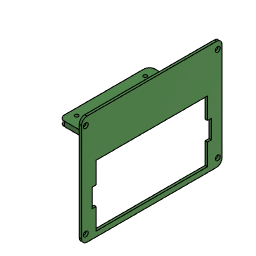
laser_module_power_control_mount v2 (Autodesk Fusion 360 design; units mm, degrees)
Autodesk Fusion 360 part; units mm, degrees
sketch "Sketch1" plane through (0, 0, 0) normal (1, 0, 0) x (0, 1, 0)
  line L0 (45, 35) -> (-45, 35)
  line L1 (-45, 35) -> (-45, -35)
  line L2 (-45, -35) -> (45, -35)
  line L3 (45, -35) -> (45, 35)
  line L4 (45, 35) -> (-45, -35) construction
  line L5 (-45, 35) -> (45, -35) construction
  line L6 (0, 0) -> (0, -35) construction
  line L7 (39.5, 9.4262) -> (-39.5, 9.4262) construction
  line L8 (-39.5, 9.4262) -> (-39.5, -33.5738) construction
  line L9 (-39.5, -33.5738) -> (39.5, -33.5738) construction
  line L10 (39.5, -33.5738) -> (39.5, 9.4262) construction
  line L11 (39.5, 9.4262) -> (-39.5, -33.5738) construction
  line L12 (-39.5, 9.4262) -> (39.5, -33.5738) construction
  line L13 (35.7, 7.5762) -> (-35.7, 7.5762)
  line L14 (-35.7, 7.5762) -> (-35.7, -31.7238)
  line L15 (-35.7, -31.7238) -> (35.7, -31.7238)
  line L16 (35.7, -31.7238) -> (35.7, 7.5762)
  line L17 (35.7, 7.5762) -> (-35.7, -31.7238) construction
  line L18 (-35.7, 7.5762) -> (35.7, -31.7238) construction
  circle A0 centre (42.2913, -30.0813) radius 1.575
  line L19 (0, 0) -> (10.5805, 0) construction
  circle A1 centre (-42.2913, -30.0813) radius 1.575
  circle A2 centre (42.2913, 30.0813) radius 1.575
  circle A3 centre (-42.2913, 30.0813) radius 1.575
  line L20 (0, 0) -> (0, 0.8708) construction
  line L21 (0, 0.8708) -> (0, 35) construction
  line L22 (25, 32.3854) -> (-25, 32.3854) construction
  line L23 (-25, 32.3854) -> (-25, 12.3854) construction
  line L24 (-25, 12.3854) -> (25, 12.3854) construction
  line L25 (25, 12.3854) -> (25, 32.3854) construction
  line L26 (25, 32.3854) -> (-25, 12.3854) construction
  line L27 (-25, 32.3854) -> (25, 12.3854) construction
  line L28 (29, 12.3854) -> (-29, 12.3854)
  line L29 (-29, 12.3854) -> (-29, 9.3854)
  line L30 (-29, 9.3854) -> (29, 9.3854)
  line L31 (29, 9.3854) -> (29, 12.3854)
  line L32 (29, 12.3854) -> (-29, 9.3854) construction
  line L33 (-29, 12.3854) -> (29, 9.3854) construction
  line L34 (0, -12.0738) -> (39.5, -12.0738) construction
  line L35 (35.7, -6.0738) -> (38.2, -6.0738)
  line L36 (38.2, -6.0738) -> (38.2, -18.0738)
  line L37 (38.2, -18.0738) -> (35.7, -18.0738)
  line L38 (35.7, -18.0738) -> (35.7, -6.0738)
  line L39 (-38.2, -18.0738) -> (-35.7, -18.0738)
  line L40 (-38.2, -6.0738) -> (-38.2, -18.0738)
  line L41 (-35.7, -6.0738) -> (-38.2, -6.0738)
  point P0 (0, -12.0738)
  point P1 (0, -12.0738)
  point P2 (0, 22.3854)
  point P3 (0, 10.8854)
  point P4 (38.2, -12.0738)
  dimension "d8" = 90
  dimension "d9" = 70
  dimension "d12" = 79
  dimension "d13" = 43
  dimension "d14" = 71.4
  dimension "d15" = 39.3
  dimension "d17" = 3.15
  dimension "d21" = 50
  dimension "d22" = 20
  dimension "d25" = 58
  dimension "d26" = 3
  dimension "d58" = 2.5
  dimension "d59" = 12
  constraint horizontal L0
  constraint perpendicular L0 L1
  constraint parallel L0 L2
  constraint parallel L1 L3
  constraint coincident L4 L6.start
  constraint coincident L5 L6.start
  constraint coincident L6.start L19.start
  constraint vertical L6
  constraint midpoint L2 L6.end
  constraint horizontal L7
  constraint perpendicular L7 L8
  constraint parallel L7 L9
  constraint parallel L8 L10
  constraint coincident L11 P1
  constraint coincident L12 P1
  constraint coincident L6 P1
  constraint horizontal L13
  constraint perpendicular L13 L14
  constraint parallel L13 L15
  constraint parallel L14 L16
  constraint coincident L17 P1
  constraint coincident L18 P1
  constraint coincident P1 P0
  constraint perpendicular L6 L19
  constraint symmetric L6 A0 A1
  constraint symmetric A0 L19 A2
  constraint symmetric L19 A1 A3
  constraint perpendicular L19 L20
  constraint midpoint L0 L21.end
  constraint perpendicular L0 L21
  constraint horizontal L22
  constraint perpendicular L22 L23
  constraint parallel L22 L24
  constraint parallel L23 L25
  constraint coincident L26 P2
  constraint coincident L27 P2
  constraint coincident L21 P2
  constraint horizontal L28
  constraint perpendicular L28 L29
  constraint parallel L28 L30
  constraint parallel L29 L31
  constraint coincident L32 P3
  constraint coincident L33 P3
  constraint coincident L21 P3
  constraint coincident L23.end L28
  constraint horizontal L34
  constraint midpoint L10 L34.end
  constraint horizontal L35
  constraint vertical L36
  constraint horizontal L37
  constraint vertical L38
  constraint coincident L16 L35.start
  constraint midpoint L36 P4
  constraint coincident L34 P4
  constraint symmetric L6 L35.start L41.start
  constraint symmetric L6 L35.end L40.start
  constraint symmetric L6 L36.end L39.start
  constraint symmetric L6 L37.end L39.end
  measures "d8" distance of L1.end L2.end
  measures "d9" distance of L0.end L1.end
  measures "d12" distance of L8.end L9.end
  measures "d13" distance of L7.end L8.end
  measures "d14" distance of L14.end L15.end
  measures "d15" distance of L13.end L14.end
  measures "d17" diameter of A0
  measures "d21" distance of L23.end L24.end
  measures "d22" distance of L22.end L23.end
  measures "d25" distance of L29.end L30.end
  measures "d26" distance of L28.end L29.end
  measures "d58" distance of L35.start L35.end
  measures "d59" distance of L35.start L37.end
extrude "Extrude1" add sketch "Sketch1" along normal blind 1.5 contours L0 L1 L2 L3 | L28 L29 L30 L31
extrude "Extrude2" add sketch "Sketch1" against normal blind 29 contours L28 L29 L30 L31
sketch "Sketch2" plane through (0, 0, 12.3854) normal (0, 0, 1) x (-1, 0, 0)
  line L0 (0, 29) -> (0, -29)
  line L1 (0, -29) -> (29, -29)
  line L2 (29, -29) -> (29, 29)
  line L3 (29, 29) -> (0, 29)
  line L4 (0, 29) -> (29, -29) construction
  line L5 (27.5, 25) -> (1.5, 25) construction
  line L6 (1.5, 25) -> (1.5, -25) construction
  line L7 (1.5, -25) -> (27.5, -25) construction
  line L8 (27.5, -25) -> (27.5, 25) construction
  line L9 (27.5, 25) -> (1.5, -25) construction
  line L10 (1.5, 25) -> (27.5, -25) construction
  circle A0 centre (4.35, -22) radius 1.575 construction
  circle A1 centre (24.65, -22) radius 1.575 construction
  circle A2 centre (4.35, 22) radius 1.575 construction
  circle A3 centre (24.65, 22) radius 1.575 construction
  line L11 (4.35, -22) -> (24.65, 22) construction
  circle A4 centre (4.35, -22) radius 1.1303
  circle A5 centre (24.65, -22) radius 1.1303
  circle A6 centre (4.35, 22) radius 1.1303
  circle A7 centre (24.65, 22) radius 1.1303
  point P0 (14.5, 0)
  point P1 (14.5, 0)
  point P2 (14.5, 0)
  dimension "d32" = 26
  dimension "d33" = 50
  dimension "d37" = 3.15
  dimension "d40" = 20.3
  dimension "d41" = 44
  dimension "d51" = 2.2606
  dimension "d54" = 20.3
  dimension "d55" = 44
  constraint coincident L0.start L3.end
  constraint coincident L1.end L2.start
  constraint midpoint L4 P2
  constraint horizontal L5
  constraint perpendicular L5 L6
  constraint parallel L5 L7
  constraint parallel L6 L8
  constraint coincident L9 P2
  constraint coincident L10 P2
  constraint coincident P2 P1
  constraint coincident A0.centre L11.start
  constraint coincident A3.centre L11.end
  constraint midpoint L11 P2
  constraint concentric A0 A4
  measures "d32" distance of L6.end L7.end
  measures "d33" distance of L5.end L6.end
  measures "d37" diameter of A0
  measures "d51" diameter of A4
fillet "Fillet1" radius 3.5 2 edges at (-29, 29, 10.8854) (-29, -29, 10.8854)
fillet "Fillet2" radius 3.5 4 edges at (0.75, 45, 35) (0.75, 45, -35) (0.75, -45, 35) (0.75, -45, -35)
sketch "Sketch3" plane through (0, -29, 0) normal (0, -1, 0) x (1, 0, 0)
  line L0 (-25.5, 12.3854) -> (-25.5, 9.3854)
  line L1 (-25.5, 9.3854) -> (0, 9.3854)
  line L2 (0, 9.3854) -> (0, 12.3854)
  line L3 (0, 12.3854) -> (-25.5, 12.3854)
  line L4 (0, 35) -> (0, -35) construction
  line L5 (-27.5, 12.3854) -> (-1.5, 12.3854) construction
  spline S0 degree 5 poles (-9.6866, 12.3854) (-9.3387, 12.3854) (-8.655, 12.4012) (-7.6662, 12.4723) (-6.4221, 12.6617) (-4.9991, 13.0566) (-3.7214, 13.6129) (-2.6063, 14.3356) (-1.6713, 15.2291) (-0.9285, 16.2912) (-0.387, 17.5173) (-0.1222, 18.6267) (-0.0222, 19.5305) (0, 20.1649) (0, 20.4901) knots 0 0 0 0 0 0 0.1 0.2 0.3 0.4 0.5 0.6 0.7 0.8 0.9 1 1 1 1 1 1
  line L6 (0, 18.6225) -> (0, 22.3578)
  line L7 (-11.558, 12.3854) -> (-7.8153, 12.3854)
  line L8 (-9.6866, 12.3854) -> (0, 12.3854)
  line L9 (0, 20.4901) -> (0, 12.3854)
  point P0 (-2.4919, 14.508)
  constraint coincident L5 S0.start
  constraint coincident L4 S0.end
  constraint midpoint S0.end L6
  constraint vertical L6
  constraint midpoint S0.start L7
  constraint horizontal L7
  constraint coincident L2.end L3.start
extrude "Extrude3" add sketch "Sketch3" against normal blind 3.5 contours L3 S0 L6 L7 L8 L9
sketch "Sketch4" plane through (0, 29, 0) normal (0, 1, 0) x (-1, 0, 0)
  line L0 (25.5, 9.3854) -> (25.5, 12.3854)
  line L1 (25.5, 12.3854) -> (0, 12.3854)
  line L2 (0, 12.3854) -> (0, 9.3854)
  line L3 (0, 9.3854) -> (25.5, 9.3854)
  line L4 (0, 12.3854) -> (9.6866, 12.3854)
  spline S0 degree 5 poles (9.6866, 12.3854) (9.3387, 12.3854) (8.655, 12.4012) (7.6662, 12.4723) (6.4221, 12.6617) (4.9991, 13.0566) (3.7214, 13.6129) (2.6063, 14.3356) (1.6713, 15.2291) (0.9285, 16.2912) (0.387, 17.5173) (0.1222, 18.6267) (0.0222, 19.5305) (0, 20.1649) (0, 20.4901) knots 0 0 0 0 0 0 0.1 0.2 0.3 0.4 0.5 0.6 0.7 0.8 0.9 1 1 1 1 1 1
  line L5 (0, 20.4901) -> (0, 12.3854)
extrude "Extrude4" add sketch "Sketch4" against normal blind 3.5 contours L1 L4 S0 L5
extrude "Extrude5" cut sketch "Sketch2" against normal blind 3 contours A4 | A5 | A6 | A7
equation "cutout_length = 71.4 mm" comment "71 mm from the manual"
equation "cutout_height = 39.3 mm" comment "39mm from the manual"
equation "plastic_thick = 1.5 mm"
equation "tab_width = 12 mm"
equation "tab_thick = 2.5 mm"
equation "panel_width = 90 mm"
equation "panel_height = 70 mm"
equation "d8 = panel_width"
equation "d9 = panel_height"
equation "power_supply_width = 79 mm"
equation "power_supply_height = 43 mm"
equation "d12 = power_supply_width"
equation "d13 = power_supply_height"
equation "d14 = cutout_length"
equation "d15 = cutout_height"
equation "mount_through_hole_diam = 3.15 mm"
equation "d17 = mount_through_hole_diam"
equation "relay_height = 20 mm"
equation "relay_length = 50 mm"
equation "relay_width = 26 mm"
equation "d21 = relay_length"
equation "d22 = relay_height"
equation "relay_ledge_thick = 3 mm"
equation "relay_ledge_length = relay_length + 8 mm"
equation "d25 = relay_ledge_length"
equation "d26 = relay_ledge_thick"
equation "relay_ledge_width = relay_width + 3 mm"
equation "d28 = plastic_thick"
equation "d30 = -relay_ledge_width"
equation "d32 = relay_width"
equation "d33 = relay_length"
equation "relay_dist_bw_holes_length = 44 mm"
equation "relay_dist_bw_holes_width = 20.3 mm"
equation "relay_hole_diam = 3.15 mm"
equation "d37 = relay_hole_diam"
equation "d40 = relay_dist_bw_holes_width"
equation "d41 = relay_dist_bw_holes_length"
equation "relay_mount_tap_diam = 0.089 in"
equation "d51 = relay_mount_tap_diam"
equation "d54 = relay_dist_bw_holes_width"
equation "d55 = relay_dist_bw_holes_length"
equation "d58 = tab_thick"
equation "d59 = tab_width"
named bodies: "laser_module_power_control_mount"
